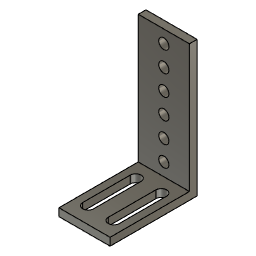
wire_guide_BOT v5 (Autodesk Fusion 360 design; units mm, degrees)
Autodesk Fusion 360 part; units mm, degrees
note: some values were not read from the file. Set by a fixed rule: which sketch regions a step uses.
sketch "Sketch1" plane through (0, 0, 0) normal (0, 1, 0) x (1, 0, 0)
  line L0 (0, 0) -> (10, 0)
  line L1 (10, 0) -> (10, -59.85)
  line L2 (10, -59.85) -> (0, -59.85)
  line L3 (0, -59.85) -> (0, 0)
  dimension "d1" = 10
  dimension "d2" = 59.85
  constraint horizontal L0
  constraint vertical L1
  constraint horizontal L2
  constraint vertical L3
  constraint coincident L0.start L3.end
  measures "d1" distance of L0.start L0.end
  measures "d2" distance of L0.start L2.end
extrude "Extrude1" add sketch "Sketch1" along normal blind 3
sketch "Sketch2" plane through (0, 0, 59.85) normal (0, 0, 1) x (-1, 0, 0)
  line L0 (0, 0) -> (-10, 0)
  line L1 (-10, 0) -> (-10, -3)
  line L2 (-10, -3) -> (0, -3)
  line L3 (0, -3) -> (0, 0)
  line L4 (0, 0) -> (-10, 0)
  line L5 (-10, 0) -> (-10, -17)
  line L6 (-10, -17) -> (0, -17)
  line L7 (0, -17) -> (0, 0)
  dimension "d5" = 17
  constraint horizontal L4
  constraint vertical L5
  constraint horizontal L6
  constraint vertical L7
  constraint coincident L0.start L3.end
  measures "d5" distance of L0.start L6.end
extrude "Extrude2" add sketch "Sketch2" along normal blind 3
sketch "Sketch3" plane through (0, 0, 62.85) normal (0, 0, 1) x (-1, 0, 0)
  line L0 (0, -17) -> (0, 0)
  line L1 (0, 0) -> (-10, 0)
  line L2 (-10, 0) -> (-10, -17)
  line L3 (-10, -17) -> (0, -17)
  line L4 (0, -3) -> (-10, -3)
  line L5 (-5, -17) -> (-5, -3) construction
  line L6 (-5, -10) -> (-5, -12.5)
  line L7 (-5, -10) -> (-5, -7.5)
  line L8 (-5, -7.5) -> (-2, -7.5)
  line L9 (-2, -7.5) -> (-2, -5.5)
  line L10 (-2, -5.5) -> (-5, -5.5)
  line L11 (-5, -5.5) -> (-5, -7.5)
  line L12 (-5, -7.5) -> (-8, -7.5)
  line L13 (-8, -7.5) -> (-8, -5.5)
  line L14 (-8, -5.5) -> (-5, -5.5)
  line L15 (-5, -10) -> (-2.0194, -10) construction
  line L16 (-5, -12.5) -> (-2, -12.5)
  line L17 (-2, -12.5) -> (-2, -14.5)
  line L18 (-2, -14.5) -> (-5, -14.5)
  line L19 (-8, -14.5) -> (-5, -14.5)
  line L20 (-8, -12.5) -> (-8, -14.5)
  line L21 (-5, -12.5) -> (-8, -12.5)
  dimension "d8" = 2.5
  dimension "d9" = 2.5
  dimension "d10" = 3
  dimension "d11" = 2
  constraint midpoint L3 L5.start
  constraint midpoint L4 L5.end
  constraint midpoint L5 L6.start
  constraint parallel L5 L6
  constraint parallel L5 L7
  constraint horizontal L8
  constraint vertical L9
  constraint horizontal L10
  constraint vertical L11
  constraint symmetric L7.end L11 L8.start
  constraint symmetric L8.end L11 L12.end
  constraint symmetric L9.end L11 L13.end
  constraint symmetric L10.end L11 L14.end
  constraint perpendicular L5 L15
  constraint symmetric L7.end L15 L6.end
  constraint symmetric L8.end L15 L16.end
  constraint symmetric L9.end L15 L17.end
  constraint symmetric L10.end L15 L18.end
  constraint symmetric L12.end L15 L20.start
  constraint symmetric L13.end L15 L19.start
  measures "d8" distance of L6.start L6.end
  measures "d9" distance of L6.start L7.end
  measures "d10" distance of L7.end L8.end
  measures "d11" distance of L7.end L10.end
extrude "Extrude3" cut sketch "Sketch3" against normal up to surface (3 mm away) contours L8 L9 L10 L11 | L11 L12 L13 L14 | L16 L17 L18 L19 L20 L21
sketch "Sketch4" plane through (0, 0, 0) normal (0, 0, -1) x (1, 0, 0)
  line L0 (10, 0) -> (0, 0)
  line L1 (0, 0) -> (0, -3)
  line L2 (0, -3) -> (10, -3)
  line L3 (10, -3) -> (10, 0)
  line L4 (0, -3) -> (10, -3)
  line L5 (10, -3) -> (10, 14)
  line L6 (10, 14) -> (0, 14)
  line L7 (0, 14) -> (0, -3)
  line L8 (5, 14) -> (5, 0) construction
  line L9 (0, 14) -> (0, 7)
  line L10 (0, 7) -> (10, 7) construction
  circle A0 centre (5, 7) radius 2
  dimension "d14" = 17
  dimension "d15" = 7
  dimension "d16" = 4
  constraint horizontal L4
  constraint vertical L5
  constraint horizontal L6
  constraint vertical L7
  constraint coincident L1.end L2.start
  constraint midpoint L6 L8.start
  constraint midpoint L0 L8.end
  constraint perpendicular L0 L8
  constraint perpendicular L6 L9
  constraint coincident L5 L10.end
  constraint perpendicular L5 L10
  constraint midpoint L10 A0.centre
  measures "d14" distance of L1.end L6.end
  measures "d15" distance of L6.end L9.end
  measures "d16" diameter of A0
extrude "Extrude4" add sketch "Sketch4" against normal blind 3 contours L0 L5 L6 L7 L9
move_face "OffsetFaces1" offset 10 1 faces at (10, 2, 20.95)
sketch "Sketch5" plane through (0, 0, 3) normal (0, 0, 1) x (-1, 0, 0)
  circle A0 centre (-5, 7) radius 2
  line L0 (-20, 14) -> (-20, 0)
  line L1 (-20, 0) -> (0, 0)
  line L2 (0, 0) -> (0, 14)
  line L3 (0, 14) -> (-20, 14)
  line L4 (-10, 14) -> (-10, 0) construction
  circle A1 centre (-15, 7) radius 2
  constraint midpoint L3 L4.start
  constraint midpoint L1 L4.end
  constraint symmetric A0 L4 A1
extrude "Extrude5" cut sketch "Sketch5" against normal up to surface (3 mm away) contours A1
sketch "Sketch6" plane through (0, 0, 0) normal (0, 0, -1) x (1, 0, 0)
  circle A0 centre (15, 7) radius 2
  circle A1 centre (5, 7) radius 2
  line L0 (0, 14) -> (0, -3)
  line L1 (0, -3) -> (20, -3)
  line L2 (20, -3) -> (20, 14)
  line L3 (20, 14) -> (0, 14)
  line L4 (-9.2754, 20.5628) -> (28.3426, 20.5628)
  line L5 (28.3426, 20.5628) -> (28.3426, -10.0286)
  line L6 (28.3426, -10.0286) -> (-9.2754, -10.0286)
  line L7 (-9.2754, -10.0286) -> (-9.2754, 20.5628)
  constraint horizontal L4
  constraint vertical L5
  constraint horizontal L6
  constraint vertical L7
extrude "Extrude6" cut sketch "Sketch6" against normal blind 9.85 contours L0 L1 L2 L3 | L4 L5 L6 L7
sketch "Sketch8" plane through (0, 0, 9.85) normal (0, 0, -1) x (1, 0, 0)
  line L0 (20, -3) -> (20, 0)
  line L1 (20, 0) -> (0, 0)
  line L2 (0, 0) -> (0, -3)
  line L3 (0, -3) -> (20, -3)
  line L4 (0, -3) -> (20, -3)
  line L5 (20, -3) -> (20, 14)
  line L6 (20, 14) -> (0, 14)
  line L7 (0, 14) -> (0, -3)
  line L8 (10, 14) -> (10, -3)
  line L9 (0, 5.9968) -> (10, 5.9968)
  circle A0 centre (5, 5.9968) radius 2
  circle A1 centre (15, 5.9968) radius 2
  dimension "d29" = 17
  dimension "d30" = 4
  constraint horizontal L4
  constraint vertical L5
  constraint horizontal L6
  constraint vertical L7
  constraint coincident L2.end L3.start
  constraint midpoint L6 L8.start
  constraint midpoint L4 L8.end
  constraint coincident L7 L9.start
  constraint coincident L8 L9.end
  constraint perpendicular L8 L9
  constraint midpoint L9 A0.centre
  constraint symmetric L8 A0 A1
  measures "d29" distance of L2.end L6.end
  measures "d30" diameter of A0
extrude "Extrude8" add sketch "Sketch8" along normal blind 3 contours L0 L1 L3 L4 L5 L8 | L1 L5 L6 L8 | L1 L2 L3 L4 L7 L8 | L1 L7 L8 L9 A0 | L6 L7 L8 L9 A0
move_face "OffsetFaces2" offset 17 1 faces at (13.3333, -14, 8.85)
sketch "Sketch9" plane through (0, 0, 6.85) normal (0, 0, -1) x (1, 0, 0)
  circle A0 centre (5, 5.9968) radius 2
  circle A1 centre (15, 5.9968) radius 2
  line L0 (0, 31) -> (0, -3)
  line L1 (0, -3) -> (20, -3)
  line L2 (20, -3) -> (20, 31)
  line L3 (20, 31) -> (0, 31)
  line L4 (0, 0) -> (20, 0) construction
  line L5 (10, 31) -> (10, 25.0709) construction
  line L6 (5, 5.9968) -> (5, 31) construction
  circle A2 centre (5, 5.9968) radius 2.125
  circle A3 centre (5, 24.5905) radius 2.125
  line L7 (5, 24.5905) -> (0, 24.5865) construction
  line L8 (5, 5.9968) -> (0, 5.9928) construction
  line L9 (2.875, 24.5888) -> (2.875, 5.9951)
  line L10 (7.125, 24.5888) -> (7.125, 5.9951)
  circle A4 centre (15, 24.5905) radius 2.125
  line L11 (12.875, 24.5888) -> (12.875, 5.9951)
  line L12 (17.125, 24.5888) -> (17.125, 5.9951)
  circle A5 centre (15, 5.9968) radius 2.125
  dimension "d51" = 4.25
  dimension "d52" = 4.25
  constraint coincident L4.start origin
  constraint coincident L2 L4.end
  constraint perpendicular L2 L4
  constraint midpoint L3 L5.start
  constraint perpendicular L3 L5
  constraint coincident A0.centre L6.start
  constraint coincident L3 L6.end
  constraint perpendicular L3 L6
  constraint coincident L6 A3.centre
  constraint coincident A3.centre L7.start
  constraint coincident L0 L7.end
  constraint coincident L0 L8.end
  constraint coincident L7 L9.start
  constraint coincident A3 L9.start
  constraint coincident L8 L9.end
  constraint coincident A2 L9.end
  constraint symmetric L6 L9.start L10.start
  constraint symmetric L6 L9.end L10.end
  constraint symmetric L5 A2 A5
  constraint symmetric L5 A3 A4
  constraint symmetric L5 L9.start L12.start
  constraint symmetric L5 L9.end L12.end
  constraint symmetric L5 L10.start L11.start
  constraint symmetric L5 L10.end L11.end
  measures "d51" diameter of A2
  measures "d52" diameter of A3
sketch "Sketch10" plane through (0, 0, 0) normal (0, -1, 0) x (1, 0, 0)
  line L0 (0, 9.85) -> (20, 9.85)
  line L1 (20, 9.85) -> (20, 62.85)
  line L2 (20, 62.85) -> (0, 62.85)
  line L3 (0, 62.85) -> (0, 9.85)
  line L4 (10, 62.85) -> (10, 9.85) construction
  circle A0 centre (10, 54.8807) radius 2
  line L5 (10, 54.8807) -> (10, 46.8807)
  circle A1 centre (10, 46.8807) radius 2
  circle A2 centre (10, 30.8807) radius 2
  circle A3 centre (10, 38.8807) radius 2
  circle A4 centre (10, 22.8807) radius 2
  circle A5 centre (10, 14.8807) radius 2
  dimension "d38" = 4
  dimension "d39" = 8
  dimension "d40" = 4
  dimension "d45" = 4
  dimension "d46" = 4
  dimension "d47" = 4
  dimension "d48" = 4
  constraint midpoint L2 L4.start
  constraint midpoint L0 L4.end
  constraint coincident L4 A0.centre
  constraint coincident A0.centre L5.start
  constraint parallel L4 L5
  constraint coincident L5.end A1.centre
  measures "d38" diameter of A0
  measures "d39" distance of A0.centre L5.end
  measures "d40" diameter of A1
  measures "d45" diameter of A3
  measures "d46" diameter of A2
  measures "d47" diameter of A4
  measures "d48" diameter of A5
extrude "Extrude10" cut sketch "Sketch10" against normal blind 3 contours A0 | A1
sketch "Sketch11" plane through (0, 0, 62.85) normal (0, 0, 1) x (-1, 0, 0)
  line L0 (-2, -12.5) -> (-2, -14.5)
  line L1 (-2, -14.5) -> (-8, -14.5)
  line L2 (-8, -14.5) -> (-8, -12.5)
  line L3 (-8, -12.5) -> (-2, -12.5)
  line L4 (-8, -7.5) -> (-8, -5.5)
  line L5 (-8, -5.5) -> (-2, -5.5)
  line L6 (-2, -5.5) -> (-2, -7.5)
  line L7 (-2, -7.5) -> (-8, -7.5)
  line L8 (0, -17) -> (0, 0)
  line L9 (0, 0) -> (-20, 0)
  line L10 (-20, 0) -> (-20, -17)
  line L11 (-20, -17) -> (0, -17)
  line L12 (5.1951, -21.2682) -> (-26.7608, -21.2682)
  line L13 (-26.7608, -21.2682) -> (-26.7608, 4.8686)
  line L14 (-26.7608, 4.8686) -> (5.1951, 4.8686)
  line L15 (5.1951, 4.8686) -> (5.1951, -21.2682)
  constraint horizontal L12
  constraint vertical L13
  constraint horizontal L14
  constraint vertical L15
extrude "Extrude11" cut sketch "Sketch11" against normal blind 3 contours L8 L9 L10 L11 | L12 L13 L14 L15
extrude "Extrude12" cut sketch "Sketch10" against normal blind 7 contours A2 | A3 | A4 | A5
extrude "Extrude13" cut sketch "Sketch9" against normal up to surface (3 mm away) contours A0 | A2 A3 L9 L10 | A3 | A4 | A4 L11 L12 A5 | A5
